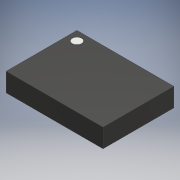
# Autodesk Inventor part: 66-0001
Saved by Autodesk Inventor 2018 (Build 220112000, 112)
## iProperties
Created: 2019-09-26
Part Number: 66-0001
Material: ABS Plastic
Document SubType Name: Modeling
Designer: Bradley
Density: 1.06 g/cm^3
Appearance: Smooth - Black
Author: Bradley
Autodesk Inventor part; units mm, degrees
ref_plane "YZ Plane" through (0, 0, 0) normal (1, 0, 0) x (0, 1, 0)
ref_plane "XZ Plane" through (0, 0, 0) normal (0, 1, 0) x (-1, 0, 0)
ref_plane "XY Plane" through (0, 0, 0) normal (0, 0, 1) x (1, 0, 0)
sketch "Sketch1" plane through (0, 0, 0) normal (0, 0, 1) x (1, 0, 0)
  line L0 (-2.6, -1.9) -> (2.6, -1.9)
  line L1 (2.6, -1.9) -> (2.6, 1.9)
  line L2 (2.6, 1.9) -> (-2.6, 1.9)
  line L3 (-2.6, 1.9) -> (-2.6, -1.9)
  line L4 (-2.6, -1.9) -> (2.6, 1.9) construction
  line L5 (2.6, -1.9) -> (-2.6, 1.9) construction
  point P0 (0, 0)
  dimension "d0" = 5.2
  dimension "d1" = 3.8
  constraints: 12 end point, 2 midpoint, 2 parallel, 1 horizontal, 1 perpendicular
  measures "d0" distance of L2.end L1.end
  measures "d1" distance of L1.end L0.end
extrude "Extrusion1" add sketch "Sketch1" along normal mid plane 1
sketch "Sketch2" plane through (0, 0, -0.5) normal (0, 0, -1) x (-1, 0, 0)
  line L0 (-2.6, -1.9) -> (2.6, -1.9) projected
  line L1 (2.6, -1.9) -> (2.6, 1.9) projected
  line L2 (2.6, 1.9) -> (-2.6, 1.9) projected
  line L3 (-2.6, 1.9) -> (-2.6, -1.9) projected
  line L4 (-2.375, 1.8) -> (-2.125, 1.8)
  line L5 (-2.125, 1.8) -> (-2.125, 1.325)
  line L6 (-2.125, 1.325) -> (-2.375, 1.325)
  line L7 (-2.375, 1.325) -> (-2.375, 1.8)
  line L8 (-2.375, -1.325) -> (-2.125, -1.325)
  line L9 (-2.125, -1.325) -> (-2.125, -1.8)
  line L10 (-2.125, -1.8) -> (-2.375, -1.8)
  line L11 (-2.375, -1.8) -> (-2.375, -1.325)
  line L12 (-2.5, 0.875) -> (-2.125, 0.875)
  line L13 (-2.125, 0.875) -> (-2.125, 0.625)
  line L14 (-2.125, 0.625) -> (-2.5, 0.625)
  line L15 (-2.5, 0.625) -> (-2.5, 0.875)
  line L16 (2.125, 0.875) -> (2.5, 0.875)
  line L17 (2.5, 0.875) -> (2.5, 0.625)
  line L18 (2.5, 0.625) -> (2.125, 0.625)
  line L19 (2.125, 0.625) -> (2.125, 0.875)
  line L20 (2.125, 0.125) -> (2.125, 0.375)
  line L21 (2.5, 0.375) -> (2.5, 0.125)
  line L22 (2.5, 0.125) -> (2.125, 0.125)
  line L23 (2.125, 0.375) -> (2.5, 0.375)
  line L24 (-2.125, 0.375) -> (-2.125, 0.125)
  line L25 (-2.5, 0.375) -> (-2.125, 0.375)
  line L26 (-2.125, 0.125) -> (-2.5, 0.125)
  line L27 (-2.5, 0.125) -> (-2.5, 0.375)
  line L28 (2.125, -0.375) -> (2.125, -0.125)
  line L29 (2.5, -0.125) -> (2.5, -0.375)
  line L30 (2.5, -0.375) -> (2.125, -0.375)
  line L31 (2.125, -0.125) -> (2.5, -0.125)
  line L32 (-2.125, -0.125) -> (-2.125, -0.375)
  line L33 (-2.5, -0.125) -> (-2.125, -0.125)
  line L34 (-2.125, -0.375) -> (-2.5, -0.375)
  line L35 (-2.5, -0.375) -> (-2.5, -0.125)
  line L36 (2.125, -0.875) -> (2.125, -0.625)
  line L37 (2.5, -0.625) -> (2.5, -0.875)
  line L38 (2.5, -0.875) -> (2.125, -0.875)
  line L39 (2.125, -0.625) -> (2.5, -0.625)
  line L40 (-2.125, -0.625) -> (-2.125, -0.875)
  line L41 (-2.5, -0.625) -> (-2.125, -0.625)
  line L42 (-2.125, -0.875) -> (-2.5, -0.875)
  line L43 (-2.5, -0.875) -> (-2.5, -0.625)
  line L44 (-1.875, -1.8) -> (-1.875, -1.325)
  line L45 (-1.625, -1.325) -> (-1.625, -1.8)
  line L46 (-1.625, -1.8) -> (-1.875, -1.8)
  line L47 (-1.875, -1.325) -> (-1.625, -1.325)
  line L48 (-1.875, 1.8) -> (-1.625, 1.8)
  line L49 (-1.625, 1.8) -> (-1.625, 1.325)
  line L50 (-1.625, 1.325) -> (-1.875, 1.325)
  line L51 (-1.875, 1.325) -> (-1.875, 1.8)
  line L52 (-1.375, -1.8) -> (-1.375, -1.325)
  line L53 (-1.125, -1.325) -> (-1.125, -1.8)
  line L54 (-1.125, -1.8) -> (-1.375, -1.8)
  line L55 (-1.375, -1.325) -> (-1.125, -1.325)
  line L56 (-1.375, 1.8) -> (-1.125, 1.8)
  line L57 (-1.125, 1.8) -> (-1.125, 1.325)
  line L58 (-1.125, 1.325) -> (-1.375, 1.325)
  line L59 (-1.375, 1.325) -> (-1.375, 1.8)
  line L60 (-0.875, -1.8) -> (-0.875, -1.325)
  line L61 (-0.625, -1.325) -> (-0.625, -1.8)
  line L62 (-0.625, -1.8) -> (-0.875, -1.8)
  line L63 (-0.875, -1.325) -> (-0.625, -1.325)
  line L64 (-0.875, 1.8) -> (-0.625, 1.8)
  line L65 (-0.625, 1.8) -> (-0.625, 1.325)
  line L66 (-0.625, 1.325) -> (-0.875, 1.325)
  line L67 (-0.875, 1.325) -> (-0.875, 1.8)
  line L68 (-0.375, -1.8) -> (-0.375, -1.325)
  line L69 (-0.125, -1.325) -> (-0.125, -1.8)
  line L70 (-0.125, -1.8) -> (-0.375, -1.8)
  line L71 (-0.375, -1.325) -> (-0.125, -1.325)
  line L72 (-0.375, 1.8) -> (-0.125, 1.8)
  line L73 (-0.125, 1.8) -> (-0.125, 1.325)
  line L74 (-0.125, 1.325) -> (-0.375, 1.325)
  line L75 (-0.375, 1.325) -> (-0.375, 1.8)
  line L76 (0.125, -1.8) -> (0.125, -1.325)
  line L77 (0.375, -1.325) -> (0.375, -1.8)
  line L78 (0.375, -1.8) -> (0.125, -1.8)
  line L79 (0.125, -1.325) -> (0.375, -1.325)
  line L80 (0.125, 1.8) -> (0.375, 1.8)
  line L81 (0.375, 1.8) -> (0.375, 1.325)
  line L82 (0.375, 1.325) -> (0.125, 1.325)
  line L83 (0.125, 1.325) -> (0.125, 1.8)
  line L84 (0.625, -1.8) -> (0.625, -1.325)
  line L85 (0.875, -1.325) -> (0.875, -1.8)
  line L86 (0.875, -1.8) -> (0.625, -1.8)
  line L87 (0.625, -1.325) -> (0.875, -1.325)
  line L88 (0.625, 1.8) -> (0.875, 1.8)
  line L89 (0.875, 1.8) -> (0.875, 1.325)
  line L90 (0.875, 1.325) -> (0.625, 1.325)
  line L91 (0.625, 1.325) -> (0.625, 1.8)
  line L92 (1.125, -1.8) -> (1.125, -1.325)
  line L93 (1.375, -1.325) -> (1.375, -1.8)
  line L94 (1.375, -1.8) -> (1.125, -1.8)
  line L95 (1.125, -1.325) -> (1.375, -1.325)
  line L96 (1.125, 1.8) -> (1.375, 1.8)
  line L97 (1.375, 1.8) -> (1.375, 1.325)
  line L98 (1.375, 1.325) -> (1.125, 1.325)
  line L99 (1.125, 1.325) -> (1.125, 1.8)
  line L100 (1.625, -1.8) -> (1.625, -1.325)
  line L101 (1.875, -1.325) -> (1.875, -1.8)
  line L102 (1.875, -1.8) -> (1.625, -1.8)
  line L103 (1.625, -1.325) -> (1.875, -1.325)
  line L104 (1.625, 1.8) -> (1.875, 1.8)
  line L105 (1.875, 1.8) -> (1.875, 1.325)
  line L106 (1.875, 1.325) -> (1.625, 1.325)
  line L107 (1.625, 1.325) -> (1.625, 1.8)
  line L108 (2.125, -1.8) -> (2.125, -1.325)
  line L109 (2.375, -1.325) -> (2.375, -1.8)
  line L110 (2.375, -1.8) -> (2.125, -1.8)
  line L111 (2.125, -1.325) -> (2.375, -1.325)
  line L112 (2.125, 1.8) -> (2.375, 1.8)
  line L113 (2.375, 1.8) -> (2.375, 1.325)
  line L114 (2.375, 1.325) -> (2.125, 1.325)
  line L115 (2.125, 1.325) -> (2.125, 1.8)
  point P0 (0, 0)
  point P1 (-2.125, 0.25)
  point P2 (-0.25, 1.325)
  dimension "d4" = 0.25
  dimension "d5" = 0.475
  dimension "d6" = 0.1
  dimension "d7" = 0.1
  dimension "d8" = 0.1
  dimension "d9" = 0.1
  dimension "d10" = 0.25
  dimension "d11" = 0.375
  dimension "d14" = 0.5
  dimension "d21" = 0.5
  dimension "d26" = 0.25
  dimension "d27" = 0.25
  constraints: 224 end point, 28 point on line, 8 parallel, 5 horizontal, 4 perpendicular, 2 collinear, 2 midpoint, 1 vertical, 192 other
  measures "d4" distance of L4.start L4.end
  measures "d5" distance of L6.end L4.start
  measures "d6" distance between parallel lines of L2 L4
  measures "d7" distance between parallel lines of L3 L15
  measures "d8" distance between parallel lines of L1 L17
  measures "d9" distance between parallel lines of L0 L10
  measures "d10" distance of L14.end L12.start
  measures "d11" distance of L12.start L12.end
  measures "d14" distance of L18.end L20.start
  measures "d21" distance of L8.start L44.end
  measures "d26" vertical distance of point (-2.125, 0.25) point (0, 0)
  measures "d27" horizontal distance of point (0, 0) point (-0.25, 1.325)
extrude "Extrusion2" add sketch "Sketch2" along normal blind 0.05 contours L4 L5 L6 L7 | L8 L9 L10 L11 | L12 L13 L14 L15 | L16 L17 L18 L19 | L20 L23 L21 L22 | L24 L26 L27 L25 | L28 L31 L29 L30 | L32 L34 L35 L33 | L36 L39 L37 L38 | L40 L42 L43 L41 | L44 L47 L45 L46 | L48 L49 L50 L51 | L52 L55 L53 L54 | L56 L57 L58 L59 | L60 L63 L61 L62 | L64 L65 L66 L67 | L68 L71 L69 L70 | L72 L73 L74 L75 | L76 L79 L77 L78 | L80 L81 L82 L83 | L84 L87 L85 L86 | L88 L89 L90 L91 | L92 L95 L93 L94 | L96 L97 L98 L99 | L100 L103 L101 L102 | L104 L105 L106 L107 | L108 L111 L109 L110 | L112 L113 L114 L115
sketch "Sketch3" plane through (0, 0, 0.5) normal (0, 0, 1) x (1, 0, 0)
  line L0 (-2.6, -1.9) -> (2.6, -1.9) projected
  line L1 (2.6, -1.9) -> (2.6, 1.9) projected
  line L2 (2.6, 1.9) -> (-2.6, 1.9) projected
  line L3 (-2.6, 1.9) -> (-2.6, -1.9) projected
  circle A0 centre (-2.1, 1.4) radius 0.5 construction
  line L4 (-2.6, 1.9) -> (2.6, 1.9) construction
  circle A1 centre (-2.1, 1.4) radius 0.25
  line L5 (-2.6, 1.9) -> (-2.6, -1.9) projected
  point P0 (0, 0)
  dimension "d30" = 0.5
  dimension "d31" = 1
  constraints: 2 centre point, 2 tangent, 1 coincident
  measures "d30" diameter of A1
  measures "d31" diameter of A0
extrude "Extrusion3" add sketch "Sketch3" along normal blind 0.01 contours A1
equation "\"d7\" = d6"
equation "\"d8\" = d7"
equation "\"d9\" = d7"
equation "\"d26\" = 0.5 * d14"
equation "\"d27\" = 0.5 * d21"
body "Solid1"
